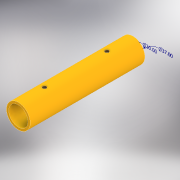
# Autodesk Inventor part: EjeRodilla
Saved by Autodesk Inventor 2021 (Build 250183000, 183)
## iProperties
Created: 2024-02-19
Part Number: EjeRodilla
Material: PLA
Document SubType Name: Modeling
Designer: Martin
Density: 1.27 g/cm^3
Appearance: PLA
Mass: 82.7781 g
Surface Area: 382.437 cm^2
Volume: 65.1796 cm^3
Author: Martin
Autodesk Inventor part; units mm, degrees
ref_plane "YZ Plane" through (0, 0, 0) normal (1, 0, 0) x (0, 1, 0)
ref_plane "XZ Plane" through (0, 0, 0) normal (0, 1, 0) x (-1, 0, 0)
sketch "Sketch1" plane through (0, 0, 0) normal (0, 0, 1) x (1, 0, 0)
  circle A0 centre (0, 0) radius 18.5
  circle A1 centre (0, 0) radius 15
  dimension "d0" = 37
  dimension "d1" = 30
  constraints: 2 centre point, 2 coincident
  measures "d0" diameter of A0
  measures "d1" diameter of A1
extrude "Extrusion1" add sketch "Sketch1" along normal mid plane 178
ref_plane "Work Plane4" through (0, 18.5, 0) normal (0, 1, 0) x (-1, 0, 0)
sketch "Sketch4" plane through (0, 18.5, 0) normal (0, 1, 0) x (-1, 0, 0)
  line L0 (-18.5, -89) -> (18.5, -89) projected
  line L1 (18.5, -89) -> (18.5, 89) projected
  line L2 (-18.5, -89) -> (18.5, -89) projected
  line L3 (18.5, 89) -> (-18.5, 89) projected
  point P0 (0, 0)
  point P1 (0, -48.5)
  dimension "d14" = 40.5
  dimension "d22" = 178
  dimension "d23" = 18.5
  constraints: 1 other
  measures "d22" distance of L1.start L1.end
  measures "d23" distance from line of L1 point (0, -48.5)
hole "Hole1" at (0, 18.5, -48.5) direction (0, -1, 0) diameter 5.9175 depth 19.1 tip angle 118 thread size "M7x1" class "6H" standard "ISO Metric profile"
mirror "Mirror1" about plane through (0, 0, 0) normal (0, 0, 1) of "Hole1"
mirror "Mirror2" about plane through (0, 0, 0) normal (0, 1, 0) of "Hole1", "Mirror1"
body "Solid1"
